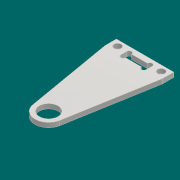
# Autodesk Inventor part: 付け根ロール_サブフレーム_6_6
Saved by Autodesk Inventor 2016 (Build 200138000, 138)
## iProperties
Created: 2016-08-24
Part Number: 付け根ロール_サブフレーム_6_6
Material: アルミニウム 2014-T4
Document SubType Name: Modeling
Designer: hiro
Density: 2.8 g/cm^3
Appearance: サテン
Mass: 4.44992 g
Surface Area: 20.0735 cm^2
Volume: 1.58926 cm^3
Author: hiro
Autodesk Inventor part; units mm, degrees
ref_plane "YZ Plane" through (0, 0, 0) normal (1, 0, 0) x (0, 1, 0)
ref_plane "XZ Plane" through (0, 0, 0) normal (0, 1, 0) x (-1, 0, 0)
ref_plane "XY Plane" through (0, 0, 0) normal (0, 0, 1) x (1, 0, 0)
derived "付け根_基準フレーム_6_1.ipt"
sketch "スケッチ1" plane through (0, 0, 0) normal (0, 0, 1) x (1, 0, 0)
  circle A0 centre (0, 0) radius 11 construction
  circle A1 centre (-13.5, -1) radius 1.35 construction
  line L0 (-13.5, -1) -> (13.5, -1) construction
  line L1 (13.5, -1) -> (13.5, -28) construction
  line L2 (13.5, -28) -> (-13.5, -28) construction
  line L3 (-13.5, -28) -> (-13.5, -1) construction
  circle A2 centre (13.5, -1) radius 1.35 construction
  circle A3 centre (-13.5, -28) radius 1.35 construction
  circle A4 centre (13.5, -28) radius 1.35 construction
  line L4 (0, 16.5) -> (0, -16.5) construction
  circle A5 centre (0, -16.5) radius 5.5 construction
  line L5 (-12.5, 27) -> (-12.5, 22)
  line L6 (-12.5, 22) -> (-5.9183, -17.4865)
  line L7 (-12.5, 27) -> (12.5, 27)
  line L8 (12.5, 27) -> (12.5, 22)
  line L9 (12.5, 22) -> (5.9183, -17.4865)
  arc A6 (-5.9183, -17.4865) -> (5.9183, -17.4865) centre (0, -16.5) ccw
  circle A7 centre (-9.5, 24.5) radius 1.55
  circle A8 centre (9.5, 24.5) radius 1.55
  line L10 (-5.55, 24.55) -> (5.55, 24.55)
  line L11 (5.55, 24.55) -> (5.55, 21.95)
  line L12 (5.55, 21.95) -> (-5.55, 21.95)
  line L13 (-5.55, 21.95) -> (-5.55, 24.55)
  circle A9 centre (-4.5, 24.55) radius 1.05
  circle A10 centre (-4.5, 21.95) radius 1.05
  circle A11 centre (4.5, 24.55) radius 1.05
  circle A12 centre (4.5, 21.95) radius 1.05
  line L14 (5.5, 24.5) -> (-5.5, 24.5) construction
  line L15 (-5.5, 24.5) -> (-5.5, 22) construction
  line L16 (-5.5, 22) -> (5.5, 22) construction
  line L17 (5.5, 22) -> (5.5, 24.5) construction
  circle A13 centre (0, -16.5) radius 4.05
  circle A14 centre (0, 8.5) radius 1.35 construction
  circle A15 centre (-8.5, 0) radius 1.35 construction
  circle A16 centre (0, -8.5) radius 1.35 construction
  circle A17 centre (8.5, 0) radius 1.35 construction
  circle A18 centre (0, 0) radius 5.05 construction
  line L18 (-9.7809, 5.0333) -> (-3.0676, 18.0786) construction
  line L19 (3.0676, 18.0786) -> (9.7809, 5.0333) construction
  arc A19 (-9.7809, 5.0333) -> (9.7809, 5.0333) centre (0, 0) ccw construction
  arc A20 (3.0676, 18.0786) -> (-3.0676, 18.0786) centre (0, 16.5) ccw construction
  circle A21 centre (0, 16.5) radius 1.55 construction
  line L20 (-10.9545, 1) -> (-14.1083, 1) construction
  line L21 (-14.1083, 1) -> (-23.805, -5.5) construction
  line L22 (-23.805, -5.5) -> (-23.805, -23.5) construction
  line L23 (-23.805, -23.5) -> (-14.1083, -30) construction
  line L24 (-14.1083, -30) -> (14.1083, -30) construction
  line L25 (14.1083, -30) -> (23.805, -23.5) construction
  line L26 (23.805, -23.5) -> (23.805, -5.5) construction
  line L27 (23.805, -5.5) -> (14.1083, 1) construction
  line L28 (14.1083, 1) -> (10.9545, 1) construction
  arc A22 (-10.9545, 1) -> (10.9545, 1) centre (0, 0) ccw construction
  line L29 (-21.755, -10.495) -> (-19.745, -10.495) construction
  line L30 (-19.745, -10.495) -> (-19.745, -18.505) construction
  line L31 (-19.745, -18.505) -> (-21.755, -18.505) construction
  line L32 (-21.755, -18.505) -> (-21.755, -10.495) construction
  line L33 (-19.75, -10.5) -> (-21.75, -10.5) construction
  line L34 (-21.75, -10.5) -> (-21.75, -18.5) construction
  line L35 (-21.75, -18.5) -> (-19.75, -18.5) construction
  line L36 (-19.75, -18.5) -> (-19.75, -10.5) construction
  circle A23 centre (-21.755, -11.545) radius 1.05 construction
  circle A24 centre (-19.745, -11.545) radius 1.05 construction
  circle A25 centre (-19.745, -17.455) radius 1.05 construction
  circle A26 centre (-21.755, -17.455) radius 1.05 construction
  circle A27 centre (-13.5, -1) radius 2 construction
  line L37 (-23.805, -14.5) -> (-19.75, -14.5) construction
  circle A28 centre (-21.755, -11.545) radius 2.05 construction
  circle A29 centre (-13.5, -28) radius 2 construction
  line L38 (21.755, -10.495) -> (19.745, -10.495) construction
  line L39 (19.75, -10.5) -> (21.75, -10.5) construction
  circle A30 centre (19.745, -11.545) radius 1.05 construction
  circle A31 centre (21.755, -11.545) radius 1.05 construction
  circle A32 centre (21.755, -11.545) radius 2.05 construction
  line L40 (23.805, -14.5) -> (19.75, -14.5) construction
  line L41 (19.75, -18.5) -> (19.75, -10.5) construction
  line L42 (21.75, -10.5) -> (21.75, -18.5) construction
  line L43 (19.745, -10.495) -> (19.745, -18.505) construction
  line L44 (21.755, -18.505) -> (21.755, -10.495) construction
  circle A33 centre (19.745, -17.455) radius 1.05 construction
  line L45 (21.75, -18.5) -> (19.75, -18.5) construction
  line L46 (19.745, -18.505) -> (21.755, -18.505) construction
  circle A34 centre (21.755, -17.455) radius 1.05 construction
  line L47 (0, -13.2668) -> (2.8, -14.8834) construction
  line L48 (2.8, -14.8834) -> (2.8, -18.1166) construction
  line L49 (2.8, -18.1166) -> (0, -19.7332) construction
  line L50 (0, -19.7332) -> (-2.8, -18.1166) construction
  line L51 (-2.8, -18.1166) -> (-2.8, -14.8834) construction
  line L52 (-2.8, -14.8834) -> (0, -13.2668) construction
  line L53 (-19.75, 12) -> (19.75, 12) construction
  line L54 (19.75, 12) -> (19.75, -39.5) construction
  line L55 (19.75, -39.5) -> (-19.75, -39.5) construction
  line L56 (-19.75, -39.5) -> (-19.75, 12) construction
  arc A35 (3.5, 16.5) -> (-3.5, 16.5) centre (0, 16.5) ccw construction
  line L57 (-3.5, 16.5) -> (-3.5, 6.8345) construction
  line L58 (3.5, 16.5) -> (3.5, 6.8345) construction
  arc A36 (-3.5, 6.8345) -> (3.5, 6.8345) centre (0, 6.8345) ccw construction
  circle A37 centre (0, 16.5) radius 5.5 construction
  line L59 (-21.75, -2) -> (-19.75, -2) construction
  line L60 (-19.75, -2) -> (-19.75, -27) construction
  line L61 (-19.75, -27) -> (-21.75, -27) construction
  line L62 (-21.75, -27) -> (-21.75, -2) construction
  circle A38 centre (0, -16.5) radius 33 construction
  line L63 (0, -16.5) -> (-23.3345, 6.8345) construction
  circle A39 centre (0, 0) radius 16.5 construction
  line L64 (-16.5, 0) -> (-23.3345, 6.8345) construction
  point P0 (0, -1)
  point P1 (0, 27)
  point P2 (-12.5, 24.5)
  point P3 (-21.75, -14.5)
extrude "押し出し1" add sketch "スケッチ1" along normal blind 2
